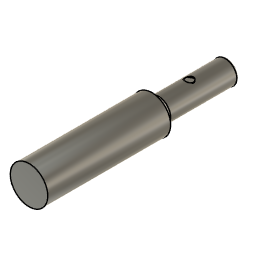
Swifter Hook v5 (Autodesk Fusion 360 design; units mm, degrees)
Autodesk Fusion 360 part; units mm, degrees
sketch "Sketch1" plane through (0, 0, 0) normal (0, 1, 0) x (1, 0, 0)
  circle A0 centre (0, 0) radius 8.636
  line L0 (-3.175, -6.35) -> (3.175, -6.35)
  line L1 (-3.175, 6.35) -> (3.175, 6.35)
  line L2 (0, -6.35) -> (0, 0) construction
  line L3 (0, 0) -> (0, 6.35) construction
  line L4 (-3.175, -6.35) -> (-3.175, -6.2217)
  line L5 (-3.175, 6.2217) -> (-3.175, 6.35)
  line L6 (3.175, -6.35) -> (3.175, -6.2217)
  line L7 (3.175, 6.2217) -> (3.175, 6.35)
  arc A1 (3.175, -6.2217) -> (3.175, 6.2217) centre (0, 0) ccw
  arc A2 (-3.175, 6.2217) -> (-3.175, -6.2217) centre (0, 0) ccw
  line L8 (3.175, 6.2217) -> (3.175, -6.2217)
  line L9 (-3.175, 6.2217) -> (-3.175, -6.2217)
  dimension "d1" = 17.272
  dimension "d2" = 13.97
  dimension "d3" = 12.7
  dimension "d4" = 6.35
  dimension "d5" = 6.35
  constraint coincident A0.centre L2.end
  constraint concentric A0 A1
  constraint horizontal L0
  constraint horizontal L1
  constraint midpoint L0 L2.start
  constraint perpendicular L1 L2
  constraint equal L0 L1
  constraint midpoint L1 L3.end
  constraint perpendicular L1 L3
  constraint coincident L5.start A1
  constraint collinear L4 L5
  constraint collinear L6 L7
  constraint concentric A1 A2
  measures "d1" diameter of A0
  measures "d2" diameter of A1
  measures "d3" distance of L0 L1
  measures "d4" distance of L0.start L0.end
  measures "d5" distance of L2.start A0.centre
extrude "Extrude1" add sketch "Sketch1" along normal blind 50.8 contours A0 | A2 L9 | A1 L8
ref_plane "WorkPlane1" through (0, 0, 9.144) normal (0, 0, 1) x (1, 0, 0)
sketch "Sketch2" plane through (0, 0, 9.144) normal (0, 0, 1) x (1, 0, 0)
  line L0 (8.636, 50.8) -> (-8.636, 50.8)
  line L1 (8.636, 0) -> (-8.636, 0)
  line L2 (8.636, 0) -> (-8.636, 0) construction
  line L3 (-8.636, 0) -> (-8.636, 22.86) construction
  line L4 (-8.636, 22.86) -> (8.636, 22.86) construction
  line L5 (8.636, 22.86) -> (8.636, 0) construction
  circle A0 centre (0, 22.86) radius 2.921
  dimension "d9" = 22.86
  dimension "d10" = 5.842
  constraint horizontal L2
  constraint vertical L3
  constraint horizontal L4
  constraint vertical L5
  constraint coincident L1.start L2.start
  constraint coincident L1.end L3
  constraint midpoint L4 A0.centre
  measures "d9" distance of L1.start L4.end
  measures "d10" diameter of A0
extrude "Extrude2" cut sketch "Sketch2" against normal through all
sketch "Sketch3" plane through (0, 0, 0) normal (0, -1, 0) x (1, 0, 0)
  line L0 (-3.175, -6.35) -> (-3.175, 6.35)
  line L1 (-3.175, 6.35) -> (3.175, 6.35)
  line L2 (3.175, 6.35) -> (3.175, -6.35)
  line L3 (3.175, -6.35) -> (-3.175, -6.35)
  circle A0 centre (0, 0) radius 8.636
  circle A1 centre (0, 0) radius 9.525
  circle A2 centre (0, 0) radius 6.985
  circle A3 centre (0, 0) radius 13.97
  dimension "d12" = 19.05
  dimension "d47" = 27.94
  constraint concentric A2 A3
  measures "d12" diameter of A1
  measures "d47" diameter of A3
extrude "Extrude3" add sketch "Sketch3" along normal blind 96.52 contours L0 L3 A2 | L0 A2 | L0 L1 L2 L3 A2 | L3 A2 | L0 L1 A2 | L2 L3 A2 | L1 A2 | L2 A2 | L1 L2 A2 | A0 | A1 | A3
ref_plane "WorkPlane2" through (-10.16, 0, 0) normal (1, 0, 0) x (0, 1, 0)
fillet "Fillet4" radius 1.27 tangency weight 2 1 edges at (-8.0516, 50.8, 3.1229)
chamfer "Chamfer3" distance 1.778 angle 45 2 edges at (-2.7233, 23.9163, -6.35) (-2.7233, 21.8037, 6.35)
chamfer "Chamfer2" distance 5.08 angle 45 1 edges at (-13.0246, 0, -5.0518)
